extrusion (Autodesk Fusion 360 design; units mm, degrees)
Autodesk Fusion 360 part; units mm, degrees
note: some values were not read from the file. Chosen so that the rebuilt part matches the saved one: which bodies a step acts on; a direction. Set by a fixed rule: which sketch regions a step uses.
sketch "Sketch1" plane through (0, 0, 0) normal (0, 1, 0) x (1, 0, 0)
  line L0 (0, 0) -> (-16, 0)
  line L1 (-16, 0) -> (-16, -1.5)
  line L2 (-16, -1.5) -> (-15.6, -1.5)
  line L3 (-15.6, -1.5) -> (-15.6, -0.4)
  line L4 (-15.6, -0.4) -> (-14.6, -0.4)
  line L5 (-14.6, -0.4) -> (-14.6, -1.5)
  line L6 (-14.6, -1.5) -> (-14.2, -1.5)
  line L7 (-14.2, -1.5) -> (-14.2, -0.4)
  line L8 (-14.2, -0.4) -> (-0.4, -0.4)
  line L9 (-0.4, -0.4) -> (-0.4, -14.2)
  line L10 (-0.4, -14.2) -> (-1.5, -14.2)
  line L11 (-1.5, -14.2) -> (-1.5, -14.6)
  line L12 (-1.5, -14.6) -> (-0.4, -14.6)
  line L13 (-0.4, -14.6) -> (-0.4, -15.6)
  line L14 (-0.4, -15.6) -> (-1.5, -15.6)
  line L15 (-1.5, -15.6) -> (-1.5, -16)
  line L16 (-1.5, -16) -> (0, -16)
  line L17 (0, -16) -> (0, 0)
  line L18 (-6.9054, -0.4) -> (-0.4, -6.9054)
  line L19 (-0.4, -7.4711) -> (-7.4711, -0.4)
  arc A0 (-16, -1.5) -> (-1.5, -16) centre (-2.2977, -2.2977) ccw
  arc A1 (-15.6, -1.5) -> (-1.5, -15.6) centre (-2.0635, -2.0635) ccw
  line L20 (-15.6, -0.4) -> (-16, -0.4)
  line L21 (-0.4, -15.6) -> (-0.4, -16)
  dimension "d1" = 16
  dimension "d2" = 16
  dimension "d3" = 0.4
  dimension "d4" = 1.5
  dimension "d5" = 0.4
  dimension "d6" = 0.4
  dimension "d7" = 1
  dimension "d9" = 0.4
  dimension "d10" = 1
  dimension "d11" = 0.4
  dimension "d12" = 0.4
  dimension "d13" = 1.5
  dimension "d15" = 45
  dimension "d16" = 10
  dimension "d17" = 0.4
  constraint coincident L0.start L17.end
  constraint horizontal L0
  constraint perpendicular L0 L1
  constraint perpendicular L1 L2
  constraint perpendicular L2 L3
  constraint perpendicular L3 L4
  constraint perpendicular L4 L5
  constraint perpendicular L5 L6
  constraint perpendicular L4 L7
  constraint perpendicular L5 L8
  constraint perpendicular L8 L9
  constraint perpendicular L9 L10
  constraint perpendicular L10 L11
  constraint perpendicular L11 L12
  constraint perpendicular L12 L13
  constraint perpendicular L11 L14
  constraint perpendicular L12 L15
  constraint perpendicular L15 L16
  constraint perpendicular L0 L17
  constraint collinear L4 L8
  constraint collinear L2 L6
  constraint collinear L9 L13
  constraint collinear L11 L15
  constraint coincident L8 L18.start
  constraint coincident L9 L18.end
  constraint coincident L9 L19.start
  constraint coincident L8 L19.end
  constraint parallel L18 L19
  constraint coincident L1 L20.end
  constraint perpendicular L1 L20
  constraint coincident L16 L21.end
  constraint perpendicular L16 L21
  measures "d1" distance of L0.start L0.end
  measures "d2" distance of L16.end L0.start
  measures "d3" distance of L0 L8
  measures "d4" distance of L0 L6
  measures "d5" distance of L1.end L2.end
  measures "d6" distance of L5.end L6.end
  measures "d7" distance of L3.end L4.end
  measures "d9" distance of L9 L17
  measures "d10" distance of L12 L14
  measures "d11" distance of L14.end L15.end
  measures "d12" distance of L10.end L11.end
  measures "d13" distance of L15.end L16.end
  measures "d15" angle of L8 L18
  measures "d16" distance of L19.start L19.end
  measures "d17" distance of L18 L19
extrude "Extrude1" add sketch "Sketch1" along normal blind 3.5 contours L0 L1 L4 L5 L6 L7 L8 L9 L10 L11 L12 L13 L16 L17 L20 L21 | L1 L2 L3 L20 | L14 L15 L16 L21 | L8 L9 L18 L19 makes body 1
extrude "Extrude2" add sketch "Sketch1" along normal blind 3.5 separate body contours L1 L2 L3 L20 | L14 L15 L16 L21 | L2 L15 A0 A1 makes body 2
sketch "Sketch2" plane through (0, 0, 0) normal (0, -1, 0) x (1, 0, 0)
  line L0 (-0.4, 0.4) -> (-6.9054, 0.4)
  line L1 (-6.9054, 0.4) -> (-0.4, 6.9054)
  line L2 (-0.4, 6.9054) -> (-0.4, 0.4)
  line L3 (-1.5, 14.2) -> (-0.4, 14.2)
  line L4 (-0.4, 14.2) -> (-0.4, 7.4711)
  line L5 (-0.4, 7.4711) -> (-7.4711, 0.4)
  line L6 (-7.4711, 0.4) -> (-14.2, 0.4)
  line L7 (-14.2, 0.4) -> (-14.2, 1.5)
  line L8 (-14.2, 1.5) -> (-14.6, 1.5)
  line L9 (-14.6, 1.5) -> (-14.6, 0.4)
  line L10 (-14.6, 0.4) -> (-15.6, 0.4)
  line L11 (-15.6, 0.4) -> (-15.6, 1.5)
  line L12 (-15.6, 1.5) -> (-16, 1.5)
  line L13 (-16, 1.5) -> (-16, 0)
  line L14 (-16, 0) -> (0, 0)
  line L15 (0, 0) -> (0, 16)
  line L16 (0, 16) -> (-1.5, 16)
  line L17 (-1.5, 16) -> (-1.5, 15.6)
  line L18 (-1.5, 15.6) -> (-0.4, 15.6)
  line L19 (-0.4, 15.6) -> (-0.4, 14.6)
  line L20 (-0.4, 14.6) -> (-1.5, 14.6)
  line L21 (-1.5, 14.6) -> (-1.5, 14.2)
  line L22 (0, 0) -> (0, 16)
  line L23 (-16, 0) -> (0, 0)
  arc A0 (0, 16) -> (-16, 0) centre (-0.4, 0.4) ccw
  line L24 (-0.4, 7.4711) -> (-0.4, 14.2)
  line L25 (-7.4711, 0.4) -> (-14.2, 0.4)
  line L26 (-0.4, 7.4711) -> (-0.4, 0.4)
  line L27 (-0.4, 0.4) -> (-7.4711, 0.4)
  line L28 (-14.2, 0.4) -> (-14.2, 1.4)
  line L29 (-7.4711, 0.4) -> (-7.4711, 1.4)
  line L30 (-7.4711, 1.4) -> (-14.2, 1.4)
  line L31 (-0.4, 14.2) -> (-1.4, 14.2)
  line L32 (-1.4, 14.2) -> (-1.4, 7.4711)
  line L33 (-1.4, 7.4711) -> (-0.4, 7.4711)
  line L34 (-7.8711, 1.4) -> (-7.8711, 0.4)
  line L35 (-13.8, 1.4) -> (-13.8, 0.4)
  line L36 (-1.4, 7.8711) -> (-0.4, 7.8711)
  line L37 (-1.4, 13.8) -> (-0.4, 13.8)
  dimension "d22" = 1
  dimension "d23" = 1
  dimension "d38" = 0.4
  dimension "d39" = 0.4
  dimension "d40" = 0.4
  dimension "d41" = 0.4
  constraint coincident L14.end L15.start
  constraint coincident L15.end L16.start
  constraint coincident L13.end L14.start
  constraint coincident L0.start L2.end
  constraint coincident L4.end L5.start
  constraint coincident L3.end L4.start
  constraint coincident L5.end L6.start
  constraint coincident L6.end L7.start
  constraint perpendicular L27 L29
  constraint perpendicular L28 L30
  constraint perpendicular L21 L31
  constraint perpendicular L31 L32
  constraint perpendicular L32 L33
  constraint coincident L30 L34.start
  constraint coincident L25 L34.end
  constraint perpendicular L25 L34
  constraint coincident L30 L35.start
  constraint coincident L25 L35.end
  constraint perpendicular L25 L35
  constraint coincident L32 L36.start
  constraint coincident L4 L36.end
  constraint perpendicular L4 L36
  constraint coincident L32 L37.start
  constraint coincident L24 L37.end
  constraint perpendicular L24 L37
  measures "d22" distance of L25 L30
  measures "d23" distance of L3.end L31.end
  measures "d38" distance of L33 L36
  measures "d39" distance of L31 L37
  measures "d40" distance of L28 L35
  measures "d41" distance of L29 L34
extrude "Extrude4" add sketch "Sketch2" against normal blind 5 separate body contours L6 L25 L30 L34 L35 | L4 L24 L32 L36 L37 makes body 3 at (-1.4, 3.3333, 11.8237) makes body 4 at (-9.8474, 3.3333, 0.4)
move_body "Move1" bodies 3 to x (1, 0, 0) y (0, 1, 0) z (0, 0, 1) at (-0.4, 0, 0.3)
move_body "Move2" bodies 4 to x (1, 0, 0) y (0, 1, 0) z (0, 0, 1) at (-0.3, 0, 0)
sketch "Sketch5" plane through (0, 0, 0) normal (1, 0, 0) x (0, 1, 0)
  line L0 (0, 16) -> (0, 0)
  line L1 (0, 0) -> (3.5, 0)
  line L2 (3.5, 0) -> (3.5, 16)
  line L3 (3.5, 16) -> (0, 16)
  arc A0 (0, 16) -> (-16, 0) centre (0, 0) ccw
  line L4 (0, 0) -> (-16, 0)
  arc A1 (0, 7.5) -> (-11, 0) centre (1.1069, -5.9402) ccw
  constraint coincident L0.start L3.end
  constraint coincident L0.end L1.start
  constraint perpendicular L0 L4
  constraint coincident L4 A1.end
  constraint coincident L0 A1.start
revolve "Revolve2" add sketch "Sketch5" angle 90 about axis through (0, 0, 0) along (0, -1, 0) contours L0 A0 L4 A1 bodies 3 4
sketch "Sketch6" plane through (-8.1832, 0, 8.1832) normal (0, -1, 0) x (1, 0, 0)
  arc A0 (5.7832, 4.7168) -> (-4.7168, -5.7832) centre (5.7832, -5.7832) ccw
  line L0 (5.7832, -5.7832) -> (5.7832, 4.7168)
  line L1 (5.7832, -5.7832) -> (-4.7168, -5.7832)
  point P0 (7.7832, -7.7832)
  dimension "d34" = 2
  dimension "d35" = 2
  dimension "d36" = 10.5
  constraint coincident A0.centre L0.start
  constraint vertical L0
  constraint perpendicular L0 L1
  measures "d34" horizontal distance of A0.centre P0
  measures "d35" distance of L1 P0
  measures "d36" radius of A0
revolve "Revolve4" cut sketch "Sketch6" angle 90 about axis through (-2.4, 0, 2.4) along (1, 0, 0) bodies 1 2 3
extrude "Extrude5" add 1 faces at (-10.1474, 1.6667, 0.4) along direction (0, 0, -1) blind 0.4 on bodies 3 bodies 3
extrude "Extrude6" cut 1 faces at (-10.1474, 1.6667, 1.4) along direction (0, 0, -1) blind 0.5 on bodies 3 bodies 3
extrude "Extrude3" [suppressed]
combine "Combine1" [suppressed]
fillet "Fillet1" [suppressed]
sketch "Sketch3" plane through (0, 0, 0) normal (1, 0, 0) x (0, 1, 0)
  spline S0 degree 3 poles (-15, 0.8541) (-15, 1.8086) (-14.9179, 2.8533) (-14.5191, 4.8961) (-14.2076, 5.8951) (-13.4847, 7.6284) (-13.0127, 8.5242) (-11.8905, 10.1964) (-11.2404, 10.9728) (-9.9324, 12.2767) (-9.1539, 12.9244) (-7.4779, 14.0413) (-6.5805, 14.5105) (-4.8737, 15.2159) (-3.907, 15.517) (-1.9318, 15.9091) (-0.9234, 16) (0, 16) knots 4.597439 4.597439 4.597439 4.597439 4.883793 4.883793 5.170148 5.170148 5.447173 5.447173 5.724199 5.724199 6.001246 6.001246 6.278292 6.278292 6.555298 6.555298 6.832304 6.832304 6.832304 6.832304
  line L0 (-15, 0.8541) -> (-15, 0)
  line L1 (-15, 0) -> (0, 0)
  line L2 (0, 0) -> (0, 16)
  line L3 (0, 7.5) -> (0, 0)
  arc A0 (0, 7.5) -> (-7.5, 0) centre (0, 0) ccw
  constraint coincident L2 L3.start
  constraint coincident L1.end L2.start
  constraint perpendicular L1 L3
  constraint coincident L1 A0.end
revolve "Revolve1" [suppressed]
hidden bodies 1 2
equation "d2 = d1"
equation "d5 = d3"
equation "d6 = d3"
equation "d9 = d3"
equation "d10 = d7"
equation "d11 = d3"
equation "d12 = d3"
equation "d13 = d4"
equation "d17 = d3"
equation "d23 = d22"
equation "d35 = d34"
equation "d39 = d38"
equation "d40 = d38"
equation "d41 = d38"
